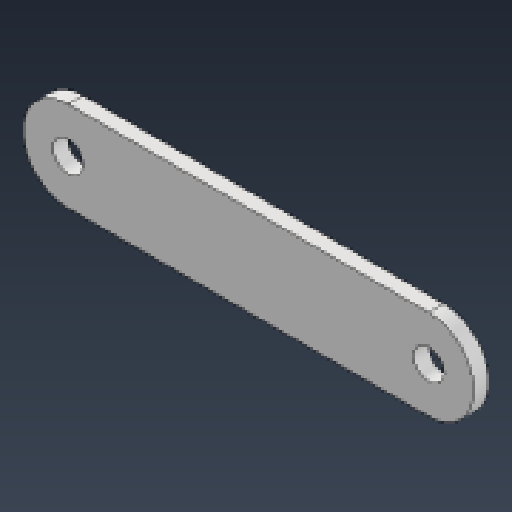
# Autodesk Inventor part: PLATE,LINK,FRONT,INTAKE
Saved by Autodesk Inventor 2026 (Build 300175050, 175E)
## iProperties
Created: 2026-02-15
Part Number: PLATE,LINK,FRONT,INTAKE
Material: Generic
Document SubType Name: Modeling
Designer: Jthib
Mass: 54.792 g
Surface Area: 211.047 cm^2
Volume: 54.792 cm^3
Density: 1 g/cm^3
Appearance: Default
Author: Jthib
Autodesk Inventor part; units mm, degrees
ref_plane "YZ Plane" through (0, 0, 0) normal (1, 0, 0) x (0, 1, 0)
ref_plane "XZ Plane" through (0, 0, 0) normal (0, 1, 0) x (-1, 0, 0)
ref_plane "XY Plane" through (0, 0, 0) normal (0, 0, 1) x (1, 0, 0)
sketch "Sketch1" plane through (0, 0, 0) normal (0, 0, 1) x (1, 0, 0)
  line L0 (-101.6, 0) -> (101.6, 0) construction
  line L1 (-101.6, -19.05) -> (101.6, -19.05)
  line L2 (101.6, 19.05) -> (-101.6, 19.05)
  arc A0 (-101.6, 19.05) -> (-101.6, -19.05) centre (-101.6, 0) ccw
  arc A1 (101.6, -19.05) -> (101.6, 19.05) centre (101.6, 0) ccw
  point P0 (0, 0)
  dimension "d1" = 38.1
  dimension "d2" = 203.2
  constraints: 8 end point, 4 point on circle, 4 tangent, 2 centre point, 1 horizontal, 1 midpoint, 1 parallel
  measures "d1" diameter of A0
  measures "d2" distance of L0.start L0.end
extrude "Extrusion1" add sketch "Sketch1" along normal mid plane 6.35
sketch "Sketch2" plane through (0, 0, 3.175) normal (0, 0, 1) x (1, 0, 0)
  arc A0 (-101.6, 19.05) -> (-101.6, -19.05) centre (-101.6, 0) ccw construction
  arc A1 (101.6, -19.05) -> (101.6, 19.05) centre (101.6, 0) ccw construction
  point P0 (0, 0)
  constraints: 2 coincident
hole "Hole1" at (-101.6, 0, 3.175) at (101.6, 0, 3.175) direction (0, 0, -1) diameter 12.7 end through all start extended yes
body "Solid1"
